Autodesk Inventor part; units mm, degrees
(part 2 of 2)
sketch "Sketch21" plane through (66.7, 15, 47.7) normal (0, 0, -1) x (-1, 0, 0)
  line L0 (7.228, 0) -> (0, 0) construction
  line L1 (0, 0) -> (0, 20) construction
  line L2 (0, 0) -> (0, 30) construction
  arc A0 (0, 20) -> (0, 30) centre (-7.7341, 25) ccw
  line L3 (0, 30) -> (0, 20)
  point P0 (66.7, -15)
  dimension "d263" = 20
  constraints: 4 end point, 2 point on circle, 1 centre point, 1 collinear, 1 point on line
  measures "d263" distance of L0.end L1.end
extrude "Extrusion19" add sketch "Sketch21" along normal mid plane 3
ref_plane "Work Plane5" through (-10, 15, -57.7) normal (-1, 0, 0) x (0, 0, 1)
ref_plane "Work Plane6" through (66.7, 15, 0) normal (0, 0, -1) x (-1, 0, 0)
mirror "Mirror3" about plane through (-10, 15, -57.7) normal (-1, 0, 0) of "Extrusion19"
mirror "Mirror4" about plane through (66.7, 15, 0) normal (0, 0, -1) of "Extrusion19", "Mirror3"
body "Solid1"
